Autodesk Fusion 360 part; units mm, degrees
(part 2 of 2)
extrude "Extrude6" cut sketch "Sketch5" against normal blind 18 contours L9 L10 A0 A1 A2 A3 | L11 L12 A4 A5 A18 A19 | L13 L14 A8 A9 A22 A23 | L15 L16 A6 A7 A20 A21 | L17 L22 A12 A13 A26 A27 | L18 L24 A10 A11 A24 A25 | L19 L21 A16 A17 A30 A31 | L20 L23 A14 A15 A28 A29
sketch "Sketch6" plane through (-2.5, 0, 0) normal (-1, 0, 0) x (0, -1, 0)
  line L0 (-2.75, 14.5) -> (-2.75, 7.5)
  line L1 (-2.75, 7.5) -> (-12.75, 7.5)
  line L2 (-12.75, 7.5) -> (-12.75, 14.5)
  line L3 (-12.75, 14.5) -> (-2.75, 14.5)
  line L4 (-30.75, 18) -> (-30.75, 21)
  line L5 (-30.75, 21) -> (-15.75, 21)
  line L6 (-15.75, 21) -> (-15.75, 18)
  line L7 (-15.75, 18) -> (-30.75, 18)
  line L8 (-73, 0) -> (2.5, 0)
  line L9 (2.5, 0) -> (2.5, 34)
  line L10 (2.5, 34) -> (-73, 34)
  line L11 (-73, 34) -> (-73, 0)
  line L12 (-73, 0) -> (-70, 0)
  line L13 (-73, 7) -> (-73, 0)
  line L14 (-41, 3) -> (-41, 31)
  line L15 (-43, 31) -> (-43, 3)
  arc A0 (-43, 3) -> (-42, 2) centre (-42, 3) ccw
  arc A1 (-42, 2) -> (-41, 3) centre (-42, 3) ccw
  arc A2 (-41, 31) -> (-42, 32) centre (-42, 31) ccw
  arc A3 (-42, 32) -> (-43, 31) centre (-42, 31) ccw
  arc A4 (-45, 31) -> (-46, 32) centre (-46, 31) ccw
  line L16 (-47, 31) -> (-47, 3)
  arc A5 (-46, 2) -> (-45, 3) centre (-46, 3) ccw
  line L17 (-45, 3) -> (-45, 31)
  arc A6 (-46, 32) -> (-47, 31) centre (-46, 31) ccw
  arc A7 (-47, 3) -> (-46, 2) centre (-46, 3) ccw
  line L18 (-53, 3) -> (-53, 31)
  line L19 (-49, 3) -> (-49, 31)
  line L20 (-55, 31) -> (-55, 3)
  arc A8 (-50, 32) -> (-51, 31) centre (-50, 31) ccw
  arc A9 (-54, 2) -> (-53, 3) centre (-54, 3) ccw
  arc A10 (-54, 32) -> (-55, 31) centre (-54, 31) ccw
  arc A11 (-53, 31) -> (-54, 32) centre (-54, 31) ccw
  line L21 (-51, 31) -> (-51, 3)
  arc A12 (-50, 2) -> (-49, 3) centre (-50, 3) ccw
  arc A13 (-49, 31) -> (-50, 32) centre (-50, 31) ccw
  arc A14 (-51, 3) -> (-50, 2) centre (-50, 3) ccw
  arc A15 (-55, 3) -> (-54, 2) centre (-54, 3) ccw
  line L22 (-63, 31) -> (-63, 3)
  arc A16 (-57, 31) -> (-58, 32) centre (-58, 31) ccw
  line L23 (-61, 3) -> (-61, 31)
  arc A17 (-59, 3) -> (-58, 2) centre (-58, 3) ccw
  arc A18 (-58, 32) -> (-59, 31) centre (-58, 31) ccw
  arc A19 (-62, 2) -> (-61, 3) centre (-62, 3) ccw
  line L24 (-57, 3) -> (-57, 31)
  arc A20 (-58, 2) -> (-57, 3) centre (-58, 3) ccw
  arc A21 (-61, 31) -> (-62, 32) centre (-62, 31) ccw
  arc A22 (-63, 3) -> (-62, 2) centre (-62, 3) ccw
  line L25 (-59, 31) -> (-59, 3)
  arc A23 (-62, 32) -> (-63, 31) centre (-62, 31) ccw
  arc A24 (-66, 32) -> (-67, 31) centre (-66, 31) ccw
  arc A25 (-67, 3) -> (-66, 2) centre (-66, 3) ccw
  line L26 (-67, 31) -> (-67, 3)
  arc A26 (-66, 2) -> (-65, 3) centre (-66, 3) ccw
  arc A27 (-65, 31) -> (-66, 32) centre (-66, 31) ccw
  line L27 (-65, 3) -> (-65, 31)
  point P0 (-41, 32)
  point P1 (-43, 2)
  point P2 (-45, 2)
  point P3 (-47, 2)
  point P4 (-45, 32)
  point P5 (-49, 2)
  point P6 (-53, 2)
  point P7 (-51, 2)
  point P8 (-49, 32)
  point P9 (-53, 32)
  point P10 (-55, 2)
  point P11 (-61, 32)
  point P12 (-57, 32)
  point P13 (-65, 32)
  dimension "d92" = 1
  dimension "d93" = 30
  dimension "d94" = 2
  dimension "d95" = 1
  dimension "d96" = 30
  dimension "d97" = 2
  dimension "d98" = 1
  dimension "d99" = 30
  dimension "d100" = 2
  dimension "d101" = 1
  dimension "d102" = 1
  dimension "d103" = 1
  dimension "d104" = 1
  constraint horizontal L12
  constraint vertical L13
  constraint coincident L8.start L11.end
  constraint coincident P1 L15
  constraint tangent L15 A0
  constraint tangent L14 A1
  constraint equal A0 A1
  constraint coincident A0.end A1.start
  constraint coincident P0 L14
  constraint tangent L14 A2
  constraint equal A0 A2
  constraint tangent L15 A3
  constraint equal A0 A3
  constraint coincident A2.end A3.start
  constraint coincident P3 L16
  constraint tangent L16 A7
  constraint coincident P2 L17
  constraint tangent A5 L17
  constraint equal A5 A7
  constraint coincident A5.start A7.end
  constraint coincident P4 L17
  constraint tangent A4 L17
  constraint equal A4 A7
  constraint tangent L16 A6
  constraint equal A6 A7
  constraint coincident A4.end A6.start
  constraint coincident P7 L21
  constraint tangent L21 A14
  constraint coincident P5 L19
  constraint tangent L19 A12
  constraint equal A12 A14
  constraint coincident A12.start A14.end
  constraint coincident P8 L19
  constraint tangent L19 A13
  constraint equal A13 A14
  constraint tangent A8 L21
  constraint equal A8 A14
  constraint coincident A8.start A13.end
  constraint coincident P10 L20
  constraint tangent L20 A15
  constraint coincident P6 L18
  constraint tangent L18 A9
  constraint equal A9 A15
  constraint coincident A9.start A15.end
  constraint coincident P9 L18
  constraint tangent L18 A11
  constraint equal A11 A15
  constraint tangent L20 A10
  constraint equal A10 A15
  constraint coincident A10.start A11.end
  constraint tangent A17 L25
  constraint tangent L24 A20
  constraint equal A17 A20
  constraint coincident A17.end A20.start
  constraint coincident P12 L24
  constraint tangent A16 L24
  constraint equal A16 A17
  constraint tangent A18 L25
  constraint equal A17 A18
  constraint coincident A16.end A18.start
  constraint tangent L22 A22
  constraint tangent L23 A19
  constraint equal A19 A22
  constraint coincident A19.start A22.end
  constraint coincident P11 L23
  constraint tangent L23 A21
  constraint equal A21 A22
  constraint tangent L22 A23
  constraint equal A22 A23
  constraint coincident A21.end A23.start
  constraint tangent A25 L26
  constraint tangent A26 L27
  constraint equal A25 A26
  constraint coincident A25.end A26.start
  constraint coincident P13 L27
  constraint tangent A27 L27
  constraint equal A25 A27
  constraint tangent A24 L26
  constraint equal A24 A25
  constraint coincident A24.start A27.end
  measures "d92" radius of A0
  measures "d93" distance of P2 P4
  measures "d94" distance of P2 P3
  measures "d95" radius of A7
  measures "d96" distance of P5 P8
  measures "d97" distance of P5 P7
  measures "d98" radius of A14
  measures "d99" distance of P6 P9
  measures "d100" distance of P6 P10
  measures "d101" radius of A15
  measures "d102" radius of A17
  measures "d103" radius of A22
  measures "d104" radius of A25
extrude "Extrude7" cut sketch "Sketch6" against normal blind 3 contours L14 L15 A0 A1 A2 A3 | A4 L16 A5 L17 A6 A7 | L18 L20 A9 A10 A11 A15 | L19 A8 L21 A12 A13 A14 | L22 L23 A19 A21 A22 A23 | A16 A17 A18 L24 A20 L25 | A24 A25 L26 A26 A27 L27
extrude "Extrude8" add 1 faces at (-1.1667, 2.75, 9.8333) along direction (0, 1, 0) blind 0.7
sketch "Sketch7" plane through (0, 0, 34) normal (0, 0, 1) x (-1, 0, 0)
  line L0 (0.5, 0.5) -> (0.5, -71)
  line L1 (0.5, -71) -> (-93, -71)
  line L2 (-93, -71) -> (-93, 0.5)
  line L3 (-93, 0.5) -> (0.5, 0.5)
  line L4 (-95, 2.5) -> (-95, -73)
  line L5 (-95, -73) -> (2.5, -73)
  line L6 (2.5, -73) -> (2.5, 2.5)
  line L7 (2.5, 2.5) -> (-95, 2.5)
  line L8 (0.5, -71) -> (-93, -71)
  line L9 (-93, -71) -> (-93, 0.5)
  line L10 (-93, 0.5) -> (0.5, 0.5)
  line L11 (0.5, 0.5) -> (0.5, -71)
  line L12 (2.5, -73) -> (-95, -73)
  line L13 (-95, -73) -> (-95, 2.5)
  line L14 (-95, 2.5) -> (2.5, 2.5)
  line L15 (2.5, 2.5) -> (2.5, -73)
  line L16 (0.5, -71) -> (2.5, -71)
  line L17 (0.5, 0.5) -> (2.5, 0.5)
  constraint horizontal L8
  constraint vertical L9
  constraint horizontal L10
  constraint vertical L11
  constraint coincident L2.end L3.start
  constraint coincident L0.end L1.start
  constraint horizontal L12
  constraint vertical L13
  constraint horizontal L14
  constraint vertical L15
  constraint coincident L4.start L7.end
  constraint coincident L5.end L6.start
  constraint coincident L6 L16.end
  constraint perpendicular L6 L16
  constraint coincident L0.start L3.end
  constraint coincident L15 L17.end
  constraint perpendicular L15 L17
extrude "Extrude9" add sketch "Sketch7" along normal blind 2 contours L1 L2 L3 L4 L5 L6 L7 L8 L9 L10 L12 L13 L14 L15 L16 L17
sketch "Sketch8" plane through (-2.5, 0, 0) normal (-1, 0, 0) x (0, -1, 0)
  line L0 (-49, 31) -> (-49, 3)
  arc A0 (-51, 3) -> (-49, 3) centre (-50, 3) ccw
  line L1 (-51, 3) -> (-51, 31)
  arc A1 (-49, 31) -> (-51, 31) centre (-50, 31) ccw
  arc A2 (-65, 31) -> (-67, 31) centre (-66, 31) ccw
  line L2 (-65, 31) -> (-65, 3)
  arc A3 (-67, 3) -> (-65, 3) centre (-66, 3) ccw
  line L3 (-67, 3) -> (-67, 31)
  line L4 (-53, 31) -> (-53, 3)
  arc A4 (-55, 3) -> (-53, 3) centre (-54, 3) ccw
  line L5 (-55, 3) -> (-55, 31)
  arc A5 (-53, 31) -> (-55, 31) centre (-54, 31) ccw
  line L6 (-45, 31) -> (-45, 3)
  arc A6 (-47, 3) -> (-45, 3) centre (-46, 3) ccw
  line L7 (-47, 3) -> (-47, 31)
  arc A7 (-45, 31) -> (-47, 31) centre (-46, 31) ccw
  line L8 (-63, 3) -> (-63, 31)
  arc A8 (-61, 31) -> (-63, 31) centre (-62, 31) ccw
  line L9 (-61, 31) -> (-61, 3)
  arc A9 (-63, 3) -> (-61, 3) centre (-62, 3) ccw
  arc A10 (-59, 3) -> (-57, 3) centre (-58, 3) ccw
  line L10 (-59, 3) -> (-59, 31)
  arc A11 (-57, 31) -> (-59, 31) centre (-58, 31) ccw
  line L11 (-57, 31) -> (-57, 3)
  line L12 (-43, 3) -> (-43, 31)
  arc A12 (-41, 31) -> (-43, 31) centre (-42, 31) ccw
  line L13 (-41, 31) -> (-41, 3)
  arc A13 (-43, 3) -> (-41, 3) centre (-42, 3) ccw
  line L14 (-3.45, 7.5) -> (-12.75, 7.5)
  line L15 (-12.75, 7.5) -> (-12.75, 14.5)
  line L16 (-12.75, 14.5) -> (-3.45, 14.5)
  line L17 (-3.45, 14.5) -> (-3.45, 7.5)
  line L18 (-30.75, 18) -> (-30.75, 21)
  line L19 (-30.75, 21) -> (-15.75, 21)
  line L20 (-15.75, 21) -> (-15.75, 18)
  line L21 (-15.75, 18) -> (-30.75, 18)
  line L22 (-73, 0) -> (2.5, 0)
  line L23 (2.5, 0) -> (2.5, 36)
  line L24 (2.5, 36) -> (0.5, 36)
  line L25 (0.5, 36) -> (0.5, 34)
  line L26 (0.5, 34) -> (-71, 34)
  line L27 (-71, 34) -> (-71, 36)
  line L28 (-71, 36) -> (-73, 36)
  line L29 (-73, 36) -> (-73, 0)
  line L30 (-71, 34) -> (-72, 34)
  line L31 (-72, 34) -> (-72, 35)
  line L32 (-72, 35) -> (-71, 35)
  line L33 (-71, 35) -> (-71, 34)
  line L34 (0.5, 34) -> (1.5, 34)
  line L35 (1.5, 34) -> (1.5, 35)
  line L36 (1.5, 35) -> (0.5, 35)
  line L37 (0.5, 35) -> (0.5, 34)
  dimension "d111" = 1
  dimension "d112" = 1
  dimension "d113" = 1
  dimension "d114" = 1
  constraint horizontal L30
  constraint vertical L31
  constraint horizontal L32
  constraint vertical L33
  constraint coincident L26.end L27.start
  constraint horizontal L34
  constraint vertical L35
  constraint horizontal L36
  constraint vertical L37
  constraint coincident L25.end L26.start
  measures "d111" distance of L31.end L32.end
  measures "d112" distance of L30.end L31.end
  measures "d113" distance of L25.end L34.end
  measures "d114" distance of L25.end L36.end
extrude "Extrude10" cut sketch "Sketch8" against normal blind 95.5 contours L27 L30 L31 L32 L33 | L25 L34 L35 L36 L37
chamfer "Chamfer2" distance 1.5 distance2 1.5 8 edges at (-2.5, 23.25, 21) (-2.5, 30.75, 19.5) (-2.5, 23.25, 18) (-2.5, 15.75, 19.5) (-2.5, 8.1, 14.5) (-2.5, 12.75, 11) (-2.5, 8.1, 7.5) (-2.5, 3.45, 11) measured on face at (-2.5, 28.1667, 9.5) measured on face at (-2.5, 28.1667, 9.5) measured on face at (-2.5, 28.1667, 9.5) measured on face at (-2.5, 28.1667, 9.5) measured on face at (-2.5, 28.1667, 9.5) measured on face at (-2.5, 28.1667, 9.5) measured on face at (-2.5, 28.1667, 9.5) measured on face at (-1.1667, 3.45, 9.8333)
extrude "Extrude11" add 1 faces at (62.5, 73, 12) along direction (0, 1, 0) blind 1
sketch "Sketch10" plane through (-2.5, 0, 0) normal (-1, 0, 0) x (0, -1, 0)
  line L0 (-32.25, 16.5) -> (-32.25, 22.5)
  line L1 (-32.25, 22.5) -> (-14.25, 22.5)
  line L2 (-14.25, 22.5) -> (-14.25, 16.5)
  line L3 (-14.25, 16.5) -> (-32.25, 16.5)
  line L4 (1.5, 34) -> (-72, 34)
  line L5 (-72, 34) -> (-72, 35)
  line L6 (-72, 35) -> (-71, 35)
  line L7 (-71, 35) -> (-71, 36)
  line L8 (-71, 36) -> (-74, 36)
  line L9 (-74, 36) -> (-74, 0)
  line L10 (-74, 0) -> (2.5, 0)
  line L11 (2.5, 0) -> (2.5, 36)
  line L12 (2.5, 36) -> (0.5, 36)
  line L13 (0.5, 36) -> (0.5, 35)
  line L14 (0.5, 35) -> (1.5, 35)
  line L15 (1.5, 35) -> (1.5, 34)
  line L16 (-49, 31) -> (-49, 3)
  arc A0 (-51, 3) -> (-49, 3) centre (-50, 3) ccw
  line L17 (-51, 3) -> (-51, 31)
  arc A1 (-49, 31) -> (-51, 31) centre (-50, 31) ccw
  arc A2 (-65, 31) -> (-67, 31) centre (-66, 31) ccw
  line L18 (-65, 31) -> (-65, 3)
  arc A3 (-67, 3) -> (-65, 3) centre (-66, 3) ccw
  line L19 (-67, 3) -> (-67, 31)
  line L20 (-53, 31) -> (-53, 3)
  arc A4 (-55, 3) -> (-53, 3) centre (-54, 3) ccw
  line L21 (-55, 3) -> (-55, 31)
  arc A5 (-53, 31) -> (-55, 31) centre (-54, 31) ccw
  line L22 (-45, 31) -> (-45, 3)
  arc A6 (-47, 3) -> (-45, 3) centre (-46, 3) ccw
  line L23 (-47, 3) -> (-47, 31)
  arc A7 (-45, 31) -> (-47, 31) centre (-46, 31) ccw
  line L24 (-63, 3) -> (-63, 31)
  arc A8 (-61, 31) -> (-63, 31) centre (-62, 31) ccw
  line L25 (-61, 31) -> (-61, 3)
  arc A9 (-63, 3) -> (-61, 3) centre (-62, 3) ccw
  arc A10 (-59, 3) -> (-57, 3) centre (-58, 3) ccw
  line L26 (-59, 3) -> (-59, 31)
  arc A11 (-57, 31) -> (-59, 31) centre (-58, 31) ccw
  line L27 (-57, 31) -> (-57, 3)
  line L28 (-43, 3) -> (-43, 31)
  arc A12 (-41, 31) -> (-43, 31) centre (-42, 31) ccw
  line L29 (-41, 31) -> (-41, 3)
  arc A13 (-43, 3) -> (-41, 3) centre (-42, 3) ccw
  line L30 (-1.95, 6) -> (-14.25, 6)
  line L31 (-14.25, 6) -> (-14.25, 16)
  line L32 (-14.25, 16) -> (-1.95, 16)
  line L33 (-1.95, 16) -> (-1.95, 6)
  line L34 (-74, 0) -> (-74, 36)
  line L35 (-74, 36) -> (-76, 36)
  line L36 (-76, 36) -> (-74, 0)
  constraint coincident L9.end L10.start
  constraint coincident L8.end L9.start
  constraint perpendicular L9 L35
extrude "Extrude12" add sketch "Sketch10" against normal blind 97.5 contours L9 L34 L35 L36
sketch "Sketch11" plane through (-2.5, 0, 0) normal (-1, 0, 0) x (0, -1, 0)
  line L0 (-32.25, 16.5) -> (-32.25, 22.5)
  line L1 (-32.25, 22.5) -> (-14.25, 22.5)
  line L2 (-14.25, 22.5) -> (-14.25, 16.5)
  line L3 (-14.25, 16.5) -> (-32.25, 16.5)
  line L4 (1.5, 34) -> (-72, 34)
  line L5 (-72, 34) -> (-72, 35)
  line L6 (-72, 35) -> (-71, 35)
  line L7 (-71, 35) -> (-71, 36)
  line L8 (-71, 36) -> (-76, 36)
  line L9 (-76, 36) -> (-74, 0)
  line L10 (-74, 0) -> (2.5, 0)
  line L11 (2.5, 0) -> (2.5, 36)
  line L12 (2.5, 36) -> (0.5, 36)
  line L13 (0.5, 36) -> (0.5, 35)
  line L14 (0.5, 35) -> (1.5, 35)
  line L15 (1.5, 35) -> (1.5, 34)
  line L16 (-49, 31) -> (-49, 3)
  arc A0 (-51, 3) -> (-49, 3) centre (-50, 3) ccw
  line L17 (-51, 3) -> (-51, 31)
  arc A1 (-49, 31) -> (-51, 31) centre (-50, 31) ccw
  arc A2 (-65, 31) -> (-67, 31) centre (-66, 31) ccw
  line L18 (-65, 31) -> (-65, 3)
  arc A3 (-67, 3) -> (-65, 3) centre (-66, 3) ccw
  line L19 (-67, 3) -> (-67, 31)
  line L20 (-53, 31) -> (-53, 3)
  arc A4 (-55, 3) -> (-53, 3) centre (-54, 3) ccw
  line L21 (-55, 3) -> (-55, 31)
  arc A5 (-53, 31) -> (-55, 31) centre (-54, 31) ccw
  line L22 (-45, 31) -> (-45, 3)
  arc A6 (-47, 3) -> (-45, 3) centre (-46, 3) ccw
  line L23 (-47, 3) -> (-47, 31)
  arc A7 (-45, 31) -> (-47, 31) centre (-46, 31) ccw
  line L24 (-63, 3) -> (-63, 31)
  arc A8 (-61, 31) -> (-63, 31) centre (-62, 31) ccw
  line L25 (-61, 31) -> (-61, 3)
  arc A9 (-63, 3) -> (-61, 3) centre (-62, 3) ccw
  arc A10 (-59, 3) -> (-57, 3) centre (-58, 3) ccw
  line L26 (-59, 3) -> (-59, 31)
  arc A11 (-57, 31) -> (-59, 31) centre (-58, 31) ccw
  line L27 (-57, 31) -> (-57, 3)
  line L28 (-43, 3) -> (-43, 31)
  arc A12 (-41, 31) -> (-43, 31) centre (-42, 31) ccw
  line L29 (-41, 31) -> (-41, 3)
  arc A13 (-43, 3) -> (-41, 3) centre (-42, 3) ccw
  line L30 (-1.95, 6) -> (-14.25, 6)
  line L31 (-14.25, 6) -> (-14.25, 16)
  line L32 (-14.25, 16) -> (-1.95, 16)
  line L33 (-1.95, 16) -> (-1.95, 6)
  line L34 (-76, 36) -> (-74.5, 36)
  line L35 (-74.5, 36) -> (-74.5, 29)
  line L36 (-74.5, 29) -> (-73, 29)
  line L37 (-73, 29) -> (-73, 36)
  line L38 (-73, 36) -> (-74.5, 36)
  dimension "d135" = 1.5
  dimension "d136" = 7
  dimension "d137" = 1.5
  constraint coincident L8.end L9.start
  constraint coincident L8 L34.end
  constraint perpendicular L8 L35
  constraint perpendicular L35 L36
  constraint coincident L8 L37.end
  constraint perpendicular L8 L37
  measures "d135" distance of L8.end L34.end
  measures "d136" distance of L34.end L35.end
  measures "d137" distance of L35.end L36.end
extrude "Extrude13" cut sketch "Sketch11" against normal blind 95.5 contours L8 L35 L36 L37 L38
sketch "Sketch12" plane through (95, 0, 0) normal (1, 0, 0) x (0, 1, 0)
  line L0 (-2.5, 0) -> (74, 0)
  line L1 (74, 0) -> (76, 36)
  line L2 (76, 36) -> (-2.5, 36)
  line L3 (-2.5, 36) -> (-2.5, 0)
  line L4 (76, 36) -> (72, 36)
  line L5 (72, 36) -> (72, 37)
  line L6 (72, 37) -> (62.5535, 90.5735)
  line L7 (72, 37) -> (126.4, 37) construction
  line L8 (72, 36) -> (-2.5, 36)
  line L9 (-2.5, 36) -> (-2.5, 90.5735)
  line L10 (-2.5, 90.5735) -> (62.5535, 90.5735)
  dimension "d140" = 4
  dimension "d141" = 1
  dimension "d142" = 100
  dimension "d143" = 54.4
  constraint coincident L1.end L2.start
  constraint coincident L2 L4.end
  constraint perpendicular L4 L5
  constraint horizontal L7
  constraint coincident L2.end L3.start
  constraint perpendicular L2 L9
  constraint perpendicular L9 L10
  measures "d140" distance of L1.end L4.end
  measures "d141" distance of L4.end L5.end
  measures "d142" angle of L6 L7
  measures "d143" distance of L5.end L6.end
extrude "Extrude14" add sketch "Sketch12" against normal blind 2 contours L2 L5 L6 L8 L9 L10
extrude "Extrude15" add 1 faces at (-1.8333, 47.1667, 34) along direction (0, 0, 1) blind 1
extrude "Extrude16" add 1 faces at (-1.1667, 23.3333, 35) along direction (0, 0, 1) blind 1
sketch "Sketch13" plane through (-2.5, 0, 0) normal (-1, 0, 0) x (0, -1, 0)
  line L0 (-1.95, 6) -> (-14.25, 6)
  line L1 (-14.25, 6) -> (-14.25, 16)
  line L2 (-14.25, 16) -> (-1.95, 16)
  line L3 (-1.95, 16) -> (-1.95, 6)
  line L4 (-43, 3) -> (-43, 31)
  arc A0 (-41, 31) -> (-43, 31) centre (-42, 31) ccw
  line L5 (-41, 31) -> (-41, 3)
  arc A1 (-43, 3) -> (-41, 3) centre (-42, 3) ccw
  arc A2 (-59, 3) -> (-57, 3) centre (-58, 3) ccw
  line L6 (-59, 3) -> (-59, 31)
  arc A3 (-57, 31) -> (-59, 31) centre (-58, 31) ccw
  line L7 (-57, 31) -> (-57, 3)
  line L8 (-63, 3) -> (-63, 31)
  arc A4 (-61, 31) -> (-63, 31) centre (-62, 31) ccw
  line L9 (-61, 31) -> (-61, 3)
  arc A5 (-63, 3) -> (-61, 3) centre (-62, 3) ccw
  line L10 (-45, 31) -> (-45, 3)
  arc A6 (-47, 3) -> (-45, 3) centre (-46, 3) ccw
  line L11 (-47, 3) -> (-47, 31)
  arc A7 (-45, 31) -> (-47, 31) centre (-46, 31) ccw
  line L12 (-53, 31) -> (-53, 3)
  arc A8 (-55, 3) -> (-53, 3) centre (-54, 3) ccw
  line L13 (-55, 3) -> (-55, 31)
  arc A9 (-53, 31) -> (-55, 31) centre (-54, 31) ccw
  arc A10 (-65, 31) -> (-67, 31) centre (-66, 31) ccw
  line L14 (-65, 31) -> (-65, 3)
  arc A11 (-67, 3) -> (-65, 3) centre (-66, 3) ccw
  line L15 (-67, 3) -> (-67, 31)
  line L16 (-49, 31) -> (-49, 3)
  arc A12 (-51, 3) -> (-49, 3) centre (-50, 3) ccw
  line L17 (-51, 3) -> (-51, 31)
  arc A13 (-49, 31) -> (-51, 31) centre (-50, 31) ccw
  line L18 (-73, 36) -> (-73, 29)
  line L19 (-73, 29) -> (-74.5, 29)
  line L20 (-74.5, 29) -> (-74.5, 36)
  line L21 (-74.5, 36) -> (-76, 36)
  line L22 (-76, 36) -> (-74, 0)
  line L23 (-74, 0) -> (2.5, 0)
  line L24 (2.5, 0) -> (2.5, 36)
  line L25 (2.5, 36) -> (-73, 36)
  line L26 (-32.25, 16.5) -> (-32.25, 22.5)
  line L27 (-32.25, 22.5) -> (-14.25, 22.5)
  line L28 (-14.25, 22.5) -> (-14.25, 16.5)
  line L29 (-14.25, 16.5) -> (-32.25, 16.5)
  line L30 (-73, 36) -> (-72, 36)
  line L31 (-72, 36) -> (-72, 37)
  line L32 (-72, 37) -> (-62.5535, 90.5735)
  line L33 (-72, 37) -> (-17.6, 37) construction
  line L34 (-72, 36) -> (2.5, 36)
  line L35 (-62.5535, 90.5735) -> (2.5, 90.5735)
  line L36 (2.5, 90.5735) -> (2.5, 36)
  dimension "d150" = 1
  dimension "d151" = 1
  dimension "d152" = 80
  dimension "d153" = 54.4
  constraint coincident L18.start L25.end
  constraint perpendicular L18 L30
  constraint perpendicular L30 L31
  constraint horizontal L33
  constraint coincident L24.end L25.start
  constraint horizontal L35
  measures "d150" distance of L18.start L30.end
  measures "d151" distance of L30.end L31.end
  measures "d152" angle of L32 L33
  measures "d153" distance of L31.end L32.end
extrude "Extrude17" add sketch "Sketch13" against normal blind 2 contours L25 L31 L32 L34 L35 L36
extrude "Extrude18" add 1 faces at (30.6667, -1.1667, 36) along direction (0, 0, 1) blind 54.5735
sketch "Sketch14" plane through (0, -2.5, 0) normal (0, -1, 0) x (1, 0, 0)
  line L0 (-2.5, 0) -> (95, 0)
  line L1 (95, 0) -> (95, 90.5735)
  line L2 (95, 90.5735) -> (93, 90.5735)
  line L3 (93, 90.5735) -> (93, 90.5735)
  line L4 (93, 90.5735) -> (-0.5, 90.5735)
  line L5 (-0.5, 90.5735) -> (-0.5, 36)
  line L6 (-0.5, 36) -> (-2.5, 36)
  line L7 (-2.5, 36) -> (-2.5, 0)
  line L8 (18.7508, 19.5) -> (18.7508, 31.5)
  line L9 (18.7508, 31.5) -> (51.2508, 31.5)
  line L10 (51.2508, 31.5) -> (51.2508, 19.5)
  line L11 (51.2508, 19.5) -> (18.7508, 19.5)
  line L12 (-0.5, 90.5735) -> (93, 90.5735)
  line L13 (93, 90.5735) -> (93, 88.5735)
  line L14 (-0.5, 90.5735) -> (-0.5, 88.5735)
  line L15 (-0.5, 88.5735) -> (93, 88.5735)
  line L16 (93, 88.5735) -> (94, 88.5735)
  line L17 (94, 88.5735) -> (94, 89.5735)
  line L18 (94, 89.5735) -> (93, 89.5735)
  line L19 (93, 89.5735) -> (93, 88.5735)
  line L20 (-0.5, 88.5735) -> (-1.5, 88.5735)
  line L21 (-1.5, 88.5735) -> (-1.5, 89.5735)
  line L22 (-1.5, 89.5735) -> (-0.5, 89.5735)
  line L23 (-0.5, 89.5735) -> (-0.5, 88.5735)
  dimension "d158" = 93.5
  dimension "d159" = 2
  dimension "d160" = 2
  dimension "d161" = 1
  dimension "d162" = 1
  dimension "d163" = 1
  dimension "d164" = 1
  constraint coincident L4.end L5.start
  constraint perpendicular L1 L12
  constraint coincident L2.end L3.start
  constraint perpendicular L4 L13
  constraint perpendicular L2 L14
  constraint horizontal L16
  constraint vertical L17
  constraint horizontal L18
  constraint vertical L19
  constraint horizontal L20
  constraint vertical L21
  constraint horizontal L22
  constraint vertical L23
  measures "d158" distance of L4.end L2.end
  measures "d159" distance of L2.end L13.end
  measures "d160" distance of L4.end L14.end
  measures "d161" distance of L13.end L16.end
  measures "d162" distance of L13.end L18.end
  measures "d163" distance of L14.end L20.end
  measures "d164" distance of L14.end L22.end
extrude "Extrude19" cut sketch "Sketch14" against normal blind 70 contours L4 L5 L12 L13 L14 L15 L19 L23 | L5 L14 L20 L21 L22 L23 | L13 L16 L17 L18 L19
sketch "Sketch15" plane through (-2.5, 0, 0) normal (-1, 0, 0) x (0, -1, 0)
  line L0 (-1.95, 6) -> (-14.25, 6)
  line L1 (-14.25, 6) -> (-14.25, 16)
  line L2 (-14.25, 16) -> (-1.95, 16)
  line L3 (-1.95, 16) -> (-1.95, 6)
  line L4 (-43, 3) -> (-43, 31)
  arc A0 (-41, 31) -> (-43, 31) centre (-42, 31) ccw
  line L5 (-41, 31) -> (-41, 3)
  arc A1 (-43, 3) -> (-41, 3) centre (-42, 3) ccw
  arc A2 (-59, 3) -> (-57, 3) centre (-58, 3) ccw
  line L6 (-59, 3) -> (-59, 31)
  arc A3 (-57, 31) -> (-59, 31) centre (-58, 31) ccw
  line L7 (-57, 31) -> (-57, 3)
  line L8 (-63, 3) -> (-63, 31)
  arc A4 (-61, 31) -> (-63, 31) centre (-62, 31) ccw
  line L9 (-61, 31) -> (-61, 3)
  arc A5 (-63, 3) -> (-61, 3) centre (-62, 3) ccw
  line L10 (-45, 31) -> (-45, 3)
  arc A6 (-47, 3) -> (-45, 3) centre (-46, 3) ccw
  line L11 (-47, 3) -> (-47, 31)
  arc A7 (-45, 31) -> (-47, 31) centre (-46, 31) ccw
  line L12 (-53, 31) -> (-53, 3)
  arc A8 (-55, 3) -> (-53, 3) centre (-54, 3) ccw
  line L13 (-55, 3) -> (-55, 31)
  arc A9 (-53, 31) -> (-55, 31) centre (-54, 31) ccw
  arc A10 (-65, 31) -> (-67, 31) centre (-66, 31) ccw
  line L14 (-65, 31) -> (-65, 3)
  arc A11 (-67, 3) -> (-65, 3) centre (-66, 3) ccw
  line L15 (-67, 3) -> (-67, 31)
  line L16 (-49, 31) -> (-49, 3)
  arc A12 (-51, 3) -> (-49, 3) centre (-50, 3) ccw
  line L17 (-51, 3) -> (-51, 31)
  arc A13 (-49, 31) -> (-51, 31) centre (-50, 31) ccw
  line L18 (-73, 36) -> (-73, 29)
  line L19 (-73, 29) -> (-74.5, 29)
  line L20 (-74.5, 29) -> (-74.5, 36)
  line L21 (-74.5, 36) -> (-76, 36)
  line L22 (-76, 36) -> (-74, 0)
  line L23 (-74, 0) -> (2.5, 0)
  line L24 (2.5, 0) -> (2.5, 36)
  line L25 (2.5, 36) -> (2.5, 90.5735)
  line L26 (2.5, 90.5735) -> (-62.5535, 90.5735)
  line L27 (-62.5535, 90.5735) -> (-72, 37)
  line L28 (-72, 37) -> (-72, 36)
  line L29 (-72, 36) -> (-73, 36)
  line L30 (-32.25, 16.5) -> (-32.25, 22.5)
  line L31 (-32.25, 22.5) -> (-14.25, 22.5)
  line L32 (-14.25, 22.5) -> (-14.25, 16.5)
  line L33 (-14.25, 16.5) -> (-32.25, 16.5)
  line L34 (-41, 31) -> (-41, 70)
  line L35 (-43, 70) -> (-43, 31)
  arc A14 (-41, 70) -> (-42, 71) centre (-42, 70) ccw
  arc A15 (-42, 71) -> (-43, 70) centre (-42, 70) ccw
  line L36 (-45, 31) -> (-45, 60)
  line L37 (-47, 31) -> (-47, 60)
  arc A16 (-46, 61) -> (-47, 60) centre (-46, 60) ccw
  arc A17 (-45, 60) -> (-46, 61) centre (-46, 60) ccw
  line L38 (-49, 31) -> (-49, 50)
  line L39 (-51, 31) -> (-51, 50)
  arc A18 (-49, 50) -> (-50, 51) centre (-50, 50) ccw
  arc A19 (-50, 51) -> (-51, 50) centre (-50, 50) ccw
  line L40 (-53, 31) -> (-53, 40)
  line L41 (-55, 31) -> (-55, 40)
  arc A20 (-53, 40) -> (-54, 41) centre (-54, 40) ccw
  arc A21 (-54, 41) -> (-55, 40) centre (-54, 40) ccw
  line L42 (-57, 31) -> (-57, 35)
  line L43 (-59, 31) -> (-59, 35)
  line L44 (-61, 31) -> (-61, 32.5)
  line L45 (-63, 31) -> (-63, 32.5)
  arc A22 (-62, 33.5) -> (-63, 32.5) centre (-62, 32.5) ccw
  arc A23 (-61, 32.5) -> (-62, 33.5) centre (-62, 32.5) ccw
  arc A24 (-58, 36) -> (-59, 35) centre (-58, 35) ccw
  arc A25 (-57, 35) -> (-58, 36) centre (-58, 35) ccw
  point P0 (-41, 71)
  point P1 (-43, 71)
  point P2 (-45, 61)
  point P3 (-47, 61)
  point P4 (-49, 51)
  point P5 (-51, 51)
  point P6 (-53, 41)
  point P7 (-55, 41)
  point P8 (-57, 36)
  point P9 (-59, 36)
  point P10 (-61, 33.5)
  point P11 (-63, 33.5)
  dimension "d167" = 40
  dimension "d168" = 2
  dimension "d169" = 1
  dimension "d170" = 30
  dimension "d171" = 30
  dimension "d172" = 1
  dimension "d173" = 20
  dimension "d174" = 20
  dimension "d175" = 1
  dimension "d176" = 10
  dimension "d177" = 10
  dimension "d178" = 1
  dimension "d179" = 5
  dimension "d180" = 5
  dimension "d181" = 2.5
  dimension "d182" = 2.5
  dimension "d183" = 1
  constraint coincident A0.start L5.start
  constraint parallel L5 L34
  constraint coincident L4.end A0.end
  constraint coincident P0 L34
  constraint tangent L34 A14
  constraint coincident P1 L35
  constraint tangent L35 A15
  constraint equal A14 A15
  constraint coincident A14.end A15.start
  constraint coincident L10.start A7.start
  constraint parallel L10 L36
  constraint coincident L11.end A7.end
  constraint parallel L11 L37
  constraint coincident P3 L37
  constraint tangent L37 A16
  constraint coincident P2 L36
  constraint tangent L36 A17
  constraint equal A16 A17
  constraint coincident A16.start A17.end
  constraint coincident L16.start A13.start
  constraint parallel L16 L38
  constraint coincident L17.end A13.end
  constraint parallel L17 L39
  constraint coincident P4 L38
  constraint tangent L38 A18
  constraint coincident P5 L39
  constraint tangent L39 A19
  constraint equal A18 A19
  constraint coincident A18.end A19.start
  constraint coincident L12.start A9.start
  constraint parallel L12 L40
  constraint coincident L13.end A9.end
  constraint parallel L13 L41
  constraint coincident P6 L40
  constraint tangent L40 A20
  constraint coincident P7 L41
  constraint tangent L41 A21
  constraint equal A20 A21
  constraint coincident A20.end A21.start
  constraint coincident A3.start L7.start
  constraint parallel L7 L42
  constraint coincident L6.end A3.end
  constraint vertical L43
  constraint coincident A4.start L9.start
  constraint coincident L8.end A4.end
  constraint parallel L8 L45
  constraint coincident P11 L45
  constraint tangent L45 A22
  constraint coincident P10 L44
  constraint tangent L44 A23
  constraint equal A22 A23
  constraint coincident A22.start A23.end
  constraint coincident P9 L43
  constraint tangent L43 A24
  constraint equal A22 A24
  constraint coincident P8 L42
  constraint tangent L42 A25
  constraint equal A22 A25
  constraint coincident A24.start A25.end
  measures "d167" distance of A0.start P0
  measures "d168" distance of P0 P1
  measures "d169" radius of A14
  measures "d170" distance of L10.start P2
  measures "d171" distance of L11.end P3
  measures "d172" radius of A16
  measures "d173" distance of L16.start P4
  measures "d174" distance of L17.end P5
  measures "d175" radius of A18
  measures "d176" distance of L12.start P6
  measures "d177" distance of L13.end P7
  measures "d178" radius of A20
  measures "d179" distance of A3.start P8
  measures "d180" distance of L6.end P9
  measures "d181" distance of A4.start P10
  measures "d182" distance of L8.end P11
  measures "d183" radius of A22
extrude "Extrude20" cut sketch "Sketch15" against normal blind 15 contours A0 L34 L35 A14 A15 | A3 L42 L43 A24 A25 | A4 L44 L45 A22 A23 | A7 L36 L37 A16 A17 | A9 L40 L41 A20 A21 | A13 L38 L39 A18 A19
equation "d48 = 5 mm + 20.5 mm"
equation "d62 = 14 mm + 5 mm"
equation "d158 = 95.5 mm - 2 mm"
